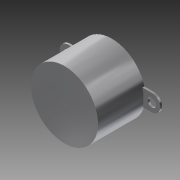
# Autodesk Inventor part: small_stepper
Saved by Autodesk Inventor 2014 (Build 180170000, 170)
## iProperties
Created: 2015-01-03
Part Number: small_stepper
Material: Bronze, Cast
Document SubType Name: Modeling
Designer: cruiser
Density: 8.87 g/cm^3
Appearance: Silver
Author: cruiser
Autodesk Inventor part; units mm, degrees
ref_plane "YZ Plane" through (0, 0, 0) normal (1, 0, 0) x (0, 1, 0)
ref_plane "XZ Plane" through (0, 0, 0) normal (0, 1, 0) x (-1, 0, 0)
ref_plane "XY Plane" through (0, 0, 0) normal (0, 0, 1) x (1, 0, 0)
sketch "Sketch1" plane through (0, 0, 0) normal (0, 1, 0) x (-1, 0, 0)
  line L0 (17.5, 0) -> (-17.5, 0) construction
  line L1 (17.5, 3.5) -> (-17.5, 3.5)
  line L2 (-17.5, -3.5) -> (17.5, -3.5)
  arc A0 (17.5, -3.5) -> (17.5, 3.5) centre (17.5, 0) ccw
  arc A1 (-17.5, 3.5) -> (-17.5, -3.5) centre (-17.5, 0) ccw
  circle A2 centre (-17.5, 0) radius 1.75
  circle A3 centre (17.5, 0) radius 1.75
  circle A4 centre (0, 0) radius 14
  dimension "d0" = 17.5
  dimension "d1" = 7
  dimension "d2" = 3.5
  dimension "d3" = 3.5
  dimension "d4" = 28
  constraints: 8 end point, 5 centre point, 4 point on circle, 4 tangent, 3 coincident, 1 horizontal, 1 midpoint, 1 parallel
  measures "d0" distance of point (0, 0) L0.end
  measures "d1" diameter of A1
  measures "d2" diameter of A2
  measures "d3" diameter of A3
  measures "d4" diameter of A4
extrude "Extrusion1" add sketch "Sketch1" against normal blind 0.8
sketch "Sketch2" plane through (0, 0, 0) normal (0, 1, 0) x (1, 0, 0)
  arc A0 (-13.5554, -3.5) -> (13.5554, -3.5) centre (0, 0) ccw projected
  line L0 (17.5, 3.5) -> (13.5554, 3.5) projected
  line L1 (0, 0) -> (0, 8)
  line L2 (0, 0) -> (8, 0) construction
  circle A1 centre (0, 8) radius 4.5
  dimension "d7" = 8
  dimension "d8" = 90
  dimension "d9" = 9
  constraints: 4 end point, 2 perpendicular, 1 centre point, 1 coincident, 1 horizontal
  measures "d7" distance of L1.start L1.end
  measures "d8" angle of L2 L1
  measures "d9" diameter of A1
extrude "Extrusion2" add sketch "Sketch2" along normal blind 1.5
sketch "Sketch3" plane through (0, 1.5, -8) normal (0, 1, 0) x (1, 0, 0)
  circle A0 centre (0, 0) radius 4.5 projected
  circle A1 centre (0, 0) radius 2.5
  point P0 (0, -8)
  dimension "d12" = 5
  constraints: 1 centre point, 1 coincident
  measures "d12" diameter of A1
extrude "Extrusion3" [suppressed]
sketch "Sketch4" plane through (0, 4, -8) normal (0, 1, 0) x (1, 0, 0)
  circle A0 centre (0, 0) radius 2.5 projected
  line L0 (2, -1.5) -> (-2, -1.5)
  line L1 (-2, -1.5) -> (-2, 1.5)
  line L2 (-2, 1.5) -> (2, 1.5)
  line L3 (2, 1.5) -> (2, -1.5)
  line L4 (2, -1.5) -> (-2, 1.5) construction
  line L5 (-2, -1.5) -> (2, 1.5) construction
  arc A1 (-2, 1.5) -> (-2, -1.5) centre (0, 0) ccw
  arc A2 (2, 1.5) -> (-2, 1.5) centre (0, 0) ccw
  arc A3 (2, -1.5) -> (2, 1.5) centre (0, 0) ccw
  arc A4 (-2, -1.5) -> (2, -1.5) centre (0, 0) ccw
  point P0 (0, -8)
  dimension "d15" = 3
  constraints: 12 end point, 8 point on circle, 4 centre point, 2 midpoint, 2 parallel, 1 coincident, 1 horizontal, 1 perpendicular, 3 other
  measures "d15" distance of L0.end L1.end
extrude "Extrusion4" [suppressed]
sketch "Sketch5" plane through (0, -0.8, 0) normal (0, -1, 0) x (1, 0, 0)
  arc A0 (13.5554, 3.5) -> (-13.5554, 3.5) centre (0, 0) ccw projected
  circle A1 centre (0, 0) radius 14
  dimension "d18" = 28
  constraints: 1 centre point, 1 coincident
  measures "d18" diameter of A1
extrude "Extrusion5" add sketch "Sketch5" along normal blind 19
equation "\"d0\" = 0.5 * stepper_screw_space"
equation "\"wood_thickness\" = 5.08"
equation "\"m3_diameter\" = 3.15"
equation "\"m5_diameter\" = 5.25"
equation "\"stepper_screw_space\" = 35"
equation "\"stepper_shaft_diameter\" = 5"
equation "\"stepper_body_diameter\" = 28"
equation "\"laser_body_diameter\" = 12"
body "Solid1"
